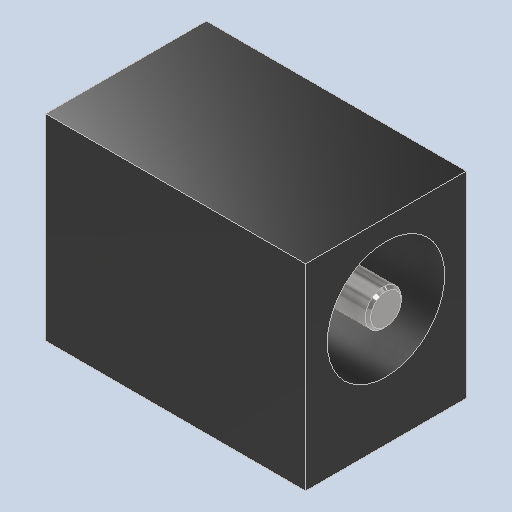
# Autodesk Inventor part: 9V_input
Saved by Autodesk Inventor 2025 (Build 290162000, 162)
## iProperties
Created: 2026-04-04
Part Number: 9V_input
Material: Polipropylen
Document SubType Name: Modeling
Designer: zzapa
Density: 0.899 g/cm^3
Appearance: Lśniąca — czarna
Author: zzapa
Autodesk Inventor part; units mm, degrees
ref_plane "YZ Plane" through (0, 0, 0) normal (1, 0, 0) x (0, 1, 0)
ref_plane "XZ Plane" through (0, 0, 0) normal (0, 1, 0) x (-1, 0, 0)
ref_plane "XY Plane" through (0, 0, 0) normal (0, 0, 1) x (1, 0, 0)
sketch "Szkic1" plane through (0, 0, 0) normal (0, 1, 0) x (-1, 0, 0)
  line L0 (14.4, -8.9) -> (0, -8.9)
  line L1 (0, -8.9) -> (0, 0)
  line L2 (0, 0) -> (14.4, 0)
  line L3 (14.4, 0) -> (14.4, -8.9)
  dimension "d0" = 8.9
  dimension "d1" = 14.4
  constraints: 8 end point, 2 parallel, 1 horizontal, 1 perpendicular
  measures "d0" distance of L2.end L0.start
  measures "d1" distance of L0.start L0.end
extrude "Wyciągnięcie proste1" add sketch "Szkic1" along normal blind 10.9
sketch "Szkic2" plane through (0, 0, 0) normal (1, 0, 0) x (0, 0, -1)
  line L0 (0, 10.9) -> (8.9, 10.9) projected
  line L1 (4.45, 10.9) -> (4.45, 0)
  line L2 (0, 0) -> (8.9, 0) projected
  circle A0 centre (4.45, 6.5) radius 1
  circle A1 centre (4.45, 6.5) radius 3.25
  dimension "d4" = 2
  dimension "d5" = 6.5
  dimension "d6" = 6.5
  constraints: 2 centre point, 2 end point, 2 midpoint, 1 coincident, 1 point on line
  measures "d4" diameter of A0
  measures "d5" diameter of A1
  measures "d6" distance from line of L2 A0.centre
extrude "Wyciągnięcie proste2" cut sketch "Szkic2" against normal blind 7 contours A1 L1 A0 | L1 A0 A1
chamfer "Faza1" distance 0.15 angle 45 1 edges at (0, 6.5, -3.45)
equation "\"d0\" = input_a"
equation "\"d1\" = input_b"
equation "\"d2\" = input_wys"
equation "\"gniazdo_M2_glebokosc\" = 1.5"
equation "\"gniazdo_M2_D1\" = 4.5"
equation "\"gniazdo_M2_D2\" = 2.6"
equation "\"insert_D\" = 2.9"
equation "\"insert_glebokosc\" = 7"
equation "\"podstawa_wys\" = 2"
equation "\"podstawa_otwory_montazowe_poz_x\" = 4"
equation "\"podstawa_otwory_montazowe_poz_y\" = 4"
equation "\"podstawa_zaokraglenie\" = 3"
equation "\"obudowa_wys\" = 45"
equation "\"obudowa_grubosc\" = 2"
equation "\"obudowa_kontrolki_a\" = 38"
equation "\"obudowa_otwory_montazowe_poz_x\" = 4"
equation "\"obudowa_otwory_montazowe_poz_y\" = 4"
equation "\"obudowa_otwory_montazowe_material_x\" = 8"
equation "\"obudowa_otwory_montazowe_material_y\" = 8"
equation "\"obudowa_zaokraglenie\" = 3"
equation "\"obudowa_otwory_io1_D\" = 12"
equation "\"obudowa_otwory_io1_wys\" = 25"
equation "\"obudowa_otwory_io1_poz\" = 55"
equation "\"obudowa_otwory_io2_D\" = 12"
equation "\"obudowa_otwory_io2_wys\" = 25"
equation "\"obudowa_otwory_io2_poz\" = 38"
equation "\"obudowa_otwory_pot_D\" = 7.2"
equation "\"input_a\" = 8.9"
equation "\"input_b\" = 14.4"
equation "\"input_wys\" = 10.9"
equation "\"obudowa_MTS_otwor_D\" = 6.2"
equation "\"obudowa_pot_poz_y\" = 15"
equation "\"obudowa_s_poz_x\" = 78"
equation "\"obudowa_s_D\" = 6.2"
equation "\"obudowa_s_poz_y\" = 15"
equation "\"obudowa_s_rozstaw_y\" = 16"
equation "\"pcb_rozstaw_x\" = 92"
equation "\"pcb_rozstaw_y\" = 58"
equation "\"obudowa_pcb_grubosc_scianki\" = 6"
equation "\"pcb_grubosc_scianki\" = 6"
equation "\"pcb_poz_y\" = 29"
equation "\"pcb_wys_bloku\" = 35"
equation "\"obudowa_footswitch_poz_y\" = 68"
equation "\"obudowa_footswitch_poz_x\" = 35"
equation "\"obudowa_footswitch_D\" = 12.3"
equation "\"obudowa_led_indicator_D\" = 3.5"
equation "\"obudowa_led_indicator_poz_x\" = 55"
equation "\"obudowa_podkladka_otwory\" = 4"
equation "\"podstawa_uchwyt_grubosc\" = 3"
equation "\"podstawa_uchwyt_wysokosc\" = 15"
equation "\"obudowa_uchwyt_grubosc\" = 2"
equation "\"pbudowa_uchwyt_podciecie_wys\" = 1.5"
equation "\"obudowa_uchwyt_wysokosc_wew\" = 26.3"
equation "\"obudowa_uchwyt_szerokosc_wew\" = 17.5"
equation "\"obudowa_gniazdo_poz\" = 25"
equation "\"obudowa_uchwyt_kolnierz_wys\" = 55"
equation "\"obudowa_uchwyt_poz_y\" = 2"
equation "\"obudowa_uchwyt_poz_z\" = 3"
equation "\"obudowa_podciecie_inout_wys\" = 6"
equation "\"obudowa_podciecie_logo_wys\" = 34"
equation "\"obudowa_podciecie_logo_szerokosc\" = 25"
equation "\"obudowa_pot_pozycjonowanie_wys\" = 13"
equation "\"obudowa_pot_pozycjonowanie_szerokosc\" = 2.8"
equation "\"obudowa_pot_pozycjonowanie_glebokosc\" = 1.4"
equation "\"obudowa_led_mocowanie_wys\" = 6"
equation "\"obudowa_led_mocowanie_poz\" = 46"
equation "\"obudowa_led_mocowanie_D\" = 5.5"
equation "\"obudowa_led_mocowanie_grubosc\" = 8"
equation "\"holder_led_grubosc\" = 2.5"
equation "\"holder_led_dlugosc\" = 28"
equation "\"holder_led_uchwyt_D\" = 5"
equation "\"holder_led_uchwyt_wysokosc\" = 5"
equation "\"holder_led_uchwyt_szerokosc\" = 8"
